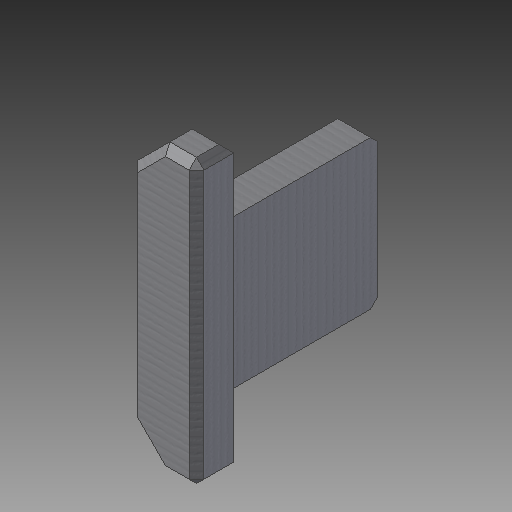
# Autodesk Inventor part: 3114a_Coil Sleeve Lock_V1
Saved by Autodesk Inventor 2020 (Build 240168000, 168)
## iProperties
Created: 2017-09-09
Part Number: 3114a_Coil Sleeve Lock_V1
Material: Acetal Resin, White
Document SubType Name: Modeling
Designer: e22ma
Density: 1.425 g/cm^3
Appearance: Smooth - White
Mass: 1.20277 g
Surface Area: 7.93303 cm^2
Volume: 0.844049 cm^3
Author: e22ma
Autodesk Inventor part; units mm, degrees
ref_plane "YZ Plane" through (0, 0, 0) normal (1, 0, 0) x (0, 1, 0)
ref_plane "Work Plane1" through (0, 0, 0) normal (0, 0, 1) x (1, 0, 0)
sketch "Sketch1" plane through (0, 0, 0) normal (0, 0, 1) x (1, 0, 0)
  line L0 (-0.2674, 6.35) -> (2.5266, 6.35)
  line L1 (2.5266, 6.35) -> (2.5266, -6.35)
  line L2 (2.9076, -6.35) -> (-0.2674, -6.35)
  line L3 (-0.2674, -6.35) -> (-0.2674, 6.35)
  line L4 (2.5266, -6.35) -> (-0.2674, -6.35)
  line L5 (-0.2674, -6.35) -> (-0.2674, 6.35)
  line L6 (-0.2674, 6.35) -> (2.5266, 6.35)
  line L7 (2.5266, 6.35) -> (2.5266, -6.35)
  point P0 (0, 0)
  dimension "d0" = 2.794
  dimension "d1" = 12.7
  constraints: 16 end point, 4 parallel, 2 horizontal, 2 perpendicular, 1 other
  measures "d0" distance between parallel lines of L3 L1
  measures "d1" distance of L2.end L0.start
extrude "Extrusion1" add sketch "Sketch1" against normal blind 12.7
ref_plane "Work Plane2" through (0, 0, 0) normal (0, 0, 1) x (1, 0, 0)
sketch "Sketch2" plane through (0, 0, 0) normal (0, 0, 1) x (1, 0, 0)
  line L0 (2.9076, -6.35) -> (-0.2674, -6.35) projected
  line L1 (-0.2674, -6.35) -> (-0.2674, 6.35) projected
  line L2 (-0.2674, 6.35) -> (2.9076, 6.35) projected
  line L3 (2.9076, 10.3713) -> (2.9076, 6.35) projected
  line L4 (2.9076, -6.35) -> (2.9076, -10.3713) projected
  line L5 (-0.2674, 6.35) -> (-0.2674, -6.35) projected
  line L6 (-0.2674, -6.35) -> (2.5266, -6.35) projected
  line L7 (2.5266, -6.35) -> (2.5266, 6.35) projected
  line L8 (2.5266, 6.35) -> (-0.2674, 6.35) projected
  line L9 (-0.2674, 6.35) -> (2.9076, 6.35)
  line L10 (2.9076, 6.35) -> (2.9076, -6.35)
  line L11 (2.9076, -6.35) -> (-0.2674, -6.35)
  line L12 (-0.2674, -6.35) -> (-0.2674, 6.35)
  line L13 (6.0826, -12.065) -> (-0.0044, -12.065) projected
  line L14 (-0.0044, 12.065) -> (6.0826, 12.065) projected
  line L15 (-2.8074, 9.262) -> (-0.0044, 12.065) projected
  line L16 (-2.8074, -9.262) -> (-2.8074, 9.262) projected
  line L17 (-0.0044, -12.065) -> (-2.8074, -9.262) projected
  line L18 (6.0826, -12.065) -> (6.0826, -10.3713) construction
  line L19 (2.9076, -10.3713) -> (6.0826, -10.3713) projected
  line L20 (6.0826, 10.3713) -> (2.9076, 10.3713) projected
  line L21 (6.0826, 10.3713) -> (6.0826, 12.065) construction
  line L22 (2.9076, -10.3713) -> (2.9076, -12.065)
  line L23 (2.9076, 10.3713) -> (2.9076, 12.065)
  point P0 (0, 0)
  constraints: 12 end point, 3 point on line, 2 parallel, 2 perpendicular, 1 horizontal
extrude "Extrusion2" add sketch "Sketch2" along normal blind 3.175
chamfer "Chamfer1" distance 0.635 angle 45 15 edges at (-1.4059, 10.6635, 3.175) (1.4516, 12.065, 3.175) (-2.8074, 0, 3.175) (-1.4059, -10.6635, 3.175) (1.4516, -12.065, 3.175) (1.4516, 12.065, 0) (1.4516, -12.065, 0) (-1.4059, -10.6635, 0) (-2.8074, 0, 0) (-1.4059, 10.6635, 0) (2.9076, 12.065, 1.5875) (2.9076, -12.065, 1.5875) (2.9076, 0, 3.175) (1.1296, 6.35, -12.7) (1.1296, -6.35, -12.7)
body "Solid1"
